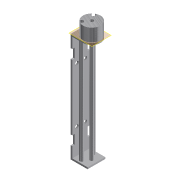
# Autodesk Inventor part: 00_Linear_Stepper_90mm
Saved by Autodesk Inventor 2022 (Build 260153000, 153)
## iProperties
Created: 2021-12-21
Part Number: 00_Linear_Stepper_90mm
Material: Generisch
Document SubType Name: Modeling
Designer: diederichbenedict
Density: 1 g/cm^3
Appearance: Maschinell bearbeitet - Aluminium
Author: diederichbenedict
Autodesk Inventor part; units mm, degrees
ref_plane "YZ Plane" through (0, 0, 0) normal (1, 0, 0) x (0, 1, 0)
ref_plane "XZ Plane" through (0, 0, 0) normal (0, 1, 0) x (-1, 0, 0)
ref_plane "XY Plane" through (0, 0, 0) normal (0, 0, 1) x (1, 0, 0)
sketch "Skizze1" plane through (0, 0, 0) normal (1, 0, 0) x (0, 1, 0)
  line L0 (0, 0) -> (-92.9, 0)
  line L1 (-92.9, 0) -> (-92.9, 15.1)
  line L2 (-92.9, 15.1) -> (0, 15.1)
  line L3 (0, 15.1) -> (0, 0)
  line L4 (-46.45, 15.1) -> (-46.45, 0)
  circle A0 centre (-69.9, 11.1) radius 1.57
  circle A1 centre (-69.9, 4) radius 1.57
  line L5 (-82.4, 15.1) -> (-74.4, 15.1)
  line L6 (-74.4, 15.1) -> (-74.4, 13.1)
  line L7 (-74.4, 13.1) -> (-82.4, 13.1)
  line L8 (-82.4, 13.1) -> (-82.4, 15.1)
  line L9 (-82.4, 0) -> (-74.4, 0)
  line L10 (-74.4, 0) -> (-74.4, 2)
  line L11 (-74.4, 2) -> (-82.4, 2)
  line L12 (-82.4, 2) -> (-82.4, 0)
  dimension "d0" = 92.9
  dimension "d1" = 15.1
  dimension "d2" = 3.14
  dimension "d3" = 3.14
  dimension "d4" = 23
  dimension "d5" = 23
  dimension "d6" = 4
  dimension "d7" = 4
  dimension "d8" = 8
  dimension "d9" = 2
  dimension "d10" = 10.5
  dimension "d11" = 2
  constraints: 26 end point, 6 parallel, 3 horizontal, 3 perpendicular, 2 centre point, 2 midpoint, 2 point on line
  measures "d0" distance of L1.end L2.end
  measures "d1" distance of L0.end L1.end
  measures "d2" diameter of A0
  measures "d3" diameter of A1
  measures "d4" distance from line of A1.centre L1
  measures "d5" distance from line of A0.centre L1
  measures "d6" distance from line of A1.centre L0
  measures "d7" distance from line of A0.centre L2
  measures "d8" distance of L6.end L7.end
  measures "d9" distance of L5.end L6.end
  measures "d10" distance between parallel lines of L8 L1
  measures "d11" distance of L10.end L9.end
extrude "Extrusion1" add sketch "Skizze1" along normal blind 1.4 contours L0 L10 L11 L12 L1 L2 L8 L7 L6 L4
mirror "Spiegeln1" about plane through (0, -46.45, 0) normal (0, 1, 0) of "Extrusion1"
sketch "Skizze2" plane through (0, -92.9, 0) normal (0, -1, 0) x (1, 0, 0)
  line L0 (0, 15.1) -> (0, 0) projected
  line L1 (0, 0) -> (1.4, 0) projected
  line L2 (1.4, 15.1) -> (1.4, 0) projected
  line L3 (0, 15.1) -> (1.4, 15.1) projected
  circle A0 centre (10.5, 7.55) radius 1.5
  circle A1 centre (6.75, 12.46) radius 1.55
  circle A2 centre (6.75, 2.64) radius 1.55
  line L4 (1.4, 15.1) -> (1.4, 13.1) projected
  line L5 (1.4, 15.1) -> (14.51, 15.1)
  line L6 (14.51, 15.1) -> (14.51, 0)
  line L7 (14.51, 0) -> (1.4, 0)
  line L8 (1.4, 0) -> (1.4, 15.1)
  dimension "d14" = 3
  dimension "d15" = 10.5
  dimension "d16" = 3.1
  dimension "d17" = 3.1
  dimension "d18" = 6.75
  dimension "d19" = 6.75
  dimension "d20" = 2.64
  dimension "d21" = 2.64
  dimension "d22" = 13.11
  constraints: 8 end point, 3 centre point, 2 parallel, 1 horizontal, 1 perpendicular
  measures "d14" diameter of A0
  measures "d15" distance from line of A0.centre L0
  measures "d16" diameter of A1
  measures "d17" diameter of A2
  measures "d18" distance from line of A1.centre L0
  measures "d19" distance from line of L0 A2.centre
  measures "d20" distance from line of A1.centre L3
  measures "d21" distance from line of A2.centre L1
  measures "d22" distance of L6.end L7.end
extrude "Extrusion2" add sketch "Skizze2" against normal blind 1.44 contours L5 L6 L7 L2
sketch "Skizze3" plane through (0, 0, 15.1) normal (0, 1, 0) x (1, 0, 0)
  line L0 (0, 0) -> (0, 15.1) projected
  line L1 (0, 0) -> (1.4, 0) projected
  line L2 (1.4, 0) -> (1.4, 15.1) projected
  line L3 (0, 15.1) -> (1.4, 15.1) projected
  line L4 (14.51, 0) -> (14.51, 15.1) projected
  line L5 (14.51, 15.1) -> (1.4, 15.1) projected
  line L6 (1.4, 0) -> (1.4, 15.1) projected
  line L7 (1.4, 0) -> (14.51, 0) projected
  circle A0 centre (10.5, 7.55) radius 1.5 projected
  circle A1 centre (6.75, 2.64) radius 1.55 projected
  circle A2 centre (6.75, 12.46) radius 1.55 projected
  circle A3 centre (10.5, 7.55) radius 7.55
  point P0 (10.5, 15.1)
  point P1 (10.5, 0)
  constraints: 1 centre point, 1 coincident, 1 tangent
extrude "Extrusion3" add sketch "Skizze3" against normal blind 1.44 contours L2 L5 A3 A2 A1 L7 | A3 A1 A2 L4 | L4 A3
ref_plane "Arbeitsebene1" through (0, 0.5, 15.1) normal (0, 1, 0) x (1, 0, 0)
sketch "Skizze4" plane through (0, 0.5, 15.1) normal (0, 1, 0) x (1, 0, 0)
  circle A0 centre (10.5, 7.55) radius 1.5 projected
  circle A1 centre (6.75, 2.64) radius 1.55 projected
  circle A2 centre (6.75, 12.46) radius 1.55 projected
  line L0 (0, 0) -> (0, 15.1) projected
  line L1 (0, 0) -> (10.5, 0) projected
  arc A3 (10.5, 0) -> (10.5, 15.1) centre (10.5, 7.55) ccw projected
  line L2 (0, 15.1) -> (10.5, 15.1) projected
  circle A4 centre (10.5, 7.55) radius 1.5 projected
  circle A5 centre (10.5, 7.55) radius 7.475
  dimension "d28" = 14.95
  constraints: 1 centre point, 1 coincident
  measures "d28" diameter of A5
extrude "Extrusion4" add sketch "Skizze4" along normal blind 10.86 contours A1 A5 A2
sketch "Skizze5" plane through (0, -91.46, 0) normal (0, 1, 0) x (1, 0, 0)
  line L0 (14.51, -15.1) -> (14.51, 0) projected
  line L1 (14.51, 0) -> (1.4, 0) projected
  line L2 (1.4, -15.1) -> (1.4, 0) projected
  line L3 (1.4, -15.1) -> (14.51, -15.1) projected
  circle A0 centre (10.5, -7.55) radius 1.5 projected
  circle A1 centre (6.75, -12.46) radius 1.55 projected
  circle A2 centre (6.75, -2.64) radius 1.55 projected
  point P0 (0, 0)
extrude "Extrusion5" add sketch "Skizze5" along normal up to surface (90.02 mm away) contours A0 | A1 | A2
equation "\"d16\" = d17"
